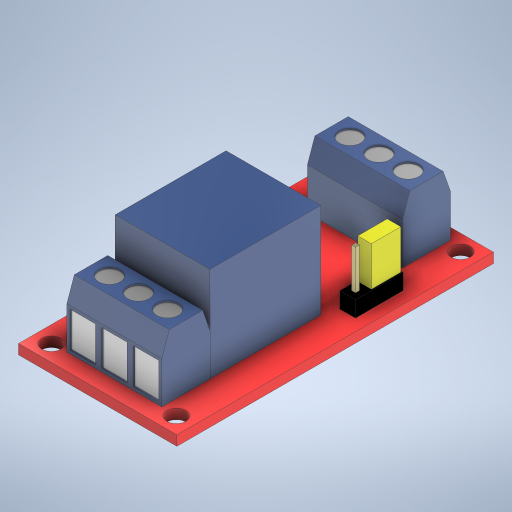
# Autodesk Inventor part: Relay
Saved by Autodesk Inventor 2024 (Build 280153000, 153)
## iProperties
Created: 2023-08-11
Part Number: Relay
Material: Generic
Document SubType Name: Modeling
Designer: 18179
Density: 1 g/cm^3
Appearance: Default
Author: 18179
Autodesk Inventor part; units mm, degrees
ref_plane "YZ Plane" through (0, 0, 0) normal (1, 0, 0) x (0, 1, 0)
ref_plane "XZ Plane" through (0, 0, 0) normal (0, 1, 0) x (-1, 0, 0)
ref_plane "XY Plane" through (0, 0, 0) normal (0, 0, 1) x (1, 0, 0)
sketch "Sketch1" plane through (0, 0, 0) normal (0, 1, 0) x (-1, 0, 0)
  line L0 (0, 0) -> (25.4, 0)
  line L1 (25.4, 0) -> (25.4, -50.8)
  line L2 (25.4, -50.8) -> (0, -50.8)
  line L3 (0, -50.8) -> (0, 0)
  line L4 (25.4, 0) -> (24.257, 0) construction
  line L5 (24.257, 0) -> (24.257, -1.143) construction
  line L6 (24.257, -1.143) -> (25.4, -1.143) construction
  line L7 (25.4, -1.143) -> (25.4, 0) construction
  line L8 (24.257, -1.143) -> (21.209, -1.143) construction
  line L9 (21.209, -1.143) -> (21.209, -4.0275) construction
  line L10 (21.209, -4.0275) -> (24.257, -4.0275) construction
  line L11 (24.257, -4.0275) -> (24.257, -1.143) construction
  line L12 (12.7, 0) -> (12.7, -12.2886) construction
  line L13 (25.4, -25.4) -> (17.1181, -25.4) construction
  circle A0 centre (22.733, -2.5852) radius 1.524
  circle A1 centre (2.667, -2.5852) radius 1.524
  circle A2 centre (22.733, -48.2148) radius 1.524
  circle A3 centre (2.667, -48.2148) radius 1.524
  dimension "d0" = 25.4
  dimension "d1" = 50.8
  dimension "d2" = 1.143
  dimension "d3" = 1.143
  dimension "d4" = 3.048
  constraints: 28 end point, 6 parallel, 4 centre point, 4 horizontal, 3 perpendicular, 3 symmetric about line, 2 midpoint, 1 vertical, 3 other
  measures "d0" distance of L1.end L2.end
  measures "d1" distance of L0.end L1.end
  measures "d2" distance of L6.end L5.end
  measures "d3" distance of L5.end L4.end
  measures "d4" distance of L10.end L9.end
extrude "Extrusion1" add sketch "Sketch1" along normal blind 1.6002
sketch "Sketch3" plane through (0, 1.6002, 0) normal (0, 1, 0) x (1, 0, 0)
  line L0 (0, 50.8) -> (-25.4, 50.8) projected
  line L1 (-12.7, 50.8) -> (-12.7, 49.022)
  line L2 (-12.7, 49.022) -> (-12.7, 41.275)
  line L3 (-25.4, 0) -> (0, 0) projected
  line L4 (-12.7, 0) -> (-12.7, 2.667)
  line L5 (-12.7, 2.667) -> (-12.7, 10.414)
  line L6 (-12.7, 10.414) -> (-5.08, 10.414)
  line L7 (-5.08, 10.414) -> (-20.32, 10.414)
  line L8 (-20.32, 10.414) -> (-20.32, 2.667)
  line L9 (-20.32, 2.667) -> (-5.08, 2.667)
  line L10 (-5.08, 2.667) -> (-5.08, 10.414)
  line L11 (-12.7, 41.275) -> (-5.08, 41.275)
  line L12 (-5.08, 41.275) -> (-5.08, 49.022)
  line L13 (-5.08, 49.022) -> (-12.7, 49.022)
  line L14 (-12.7, 49.022) -> (-12.7, 41.275)
  line L15 (-5.08, 41.275) -> (-20.32, 41.275)
  line L16 (-20.32, 41.275) -> (-20.32, 49.022)
  line L17 (-20.32, 49.022) -> (-5.08, 49.022)
  line L18 (-5.08, 49.022) -> (-5.08, 41.275)
  dimension "d13" = 7.747
  dimension "d14" = 1.778
  dimension "d15" = 2.667
  dimension "d16" = 7.747
  dimension "d17" = 7.62
  dimension "d18" = 15.24
  dimension "d19" = 7.747
  dimension "d20" = 7.62
  dimension "d21" = 7.747
  dimension "d22" = 15.24
  constraints: 34 end point, 6 parallel, 4 perpendicular, 3 horizontal, 3 point on line, 2 midpoint, 2 vertical
  measures "d13" distance of L1.end L2.end
  measures "d14" distance of L1.start L1.end
  measures "d15" distance of L4.start L4.end
  measures "d16" distance of L4.end L5.end
  measures "d17" distance of L5.end L6.end
  measures "d18" distance of L9.end L8.end
  measures "d19" distance of L8.end L7.end
  measures "d20" distance of L13.end L12.end
  measures "d21" distance of L12.end L11.end
  measures "d22" distance of L16.end L17.end
extrude "Extrusion2" add sketch "Sketch3" along normal blind 10.16
chamfer "Chamfer1" distance 1.1938 distance2 3.429 2 edges at (-12.7, 11.7602, -2.667) (-12.7, 11.7602, -10.414) measured on face at (-12.7, 11.7602, -9.914) measured on face at (-12.7, 11.7602, -3.167)
chamfer "Chamfer2" distance 1.1938 distance2 3.429 2 edges at (-12.7, 11.7602, -41.275) (-12.7, 11.7602, -49.022) measured on face at (-12.7, 11.7602, -48.522) measured on face at (-12.7, 11.7602, -41.775)
sketch "Sketch4" plane through (0, 11.7602, 0) normal (0, 1, 0) x (1, 0, 0)
  line L0 (-5.08, 42.4688) -> (-20.32, 42.4688) projected
  line L1 (-20.32, 41.275) -> (-20.32, 49.022) projected
  line L2 (-5.08, 42.4688) -> (-20.32, 42.4688)
  line L3 (-20.32, 42.4688) -> (-20.32, 45.1485)
  line L4 (-20.32, 45.1485) -> (-5.08, 45.1485)
  line L5 (-5.08, 45.1485) -> (-5.08, 42.4688)
  circle A0 centre (-12.7, 45.1485) radius 1.7145
  line L6 (-10.9855, 45.1485) -> (-5.08, 45.1485)
  line L7 (-5.08, 49.022) -> (-5.08, 41.275) projected
  line L8 (-14.4145, 45.1485) -> (-20.32, 45.1485)
  line L9 (-5.08, 3.8608) -> (-20.32, 3.8608) projected
  line L10 (-20.32, 2.667) -> (-20.32, 10.414) projected
  line L11 (-5.08, 3.8608) -> (-20.32, 3.8608)
  line L12 (-20.32, 3.8608) -> (-20.32, 6.5405)
  line L13 (-20.32, 6.5405) -> (-5.08, 6.5405)
  line L14 (-5.08, 6.5405) -> (-5.08, 3.8608)
  circle A1 centre (-8.0328, 45.1485) radius 1.7145
  circle A2 centre (-17.3672, 45.1485) radius 1.7145
  circle A3 centre (-12.7, 6.5405) radius 1.7145
  line L15 (-10.9855, 6.5405) -> (-5.08, 6.5405)
  line L16 (-14.4145, 6.5405) -> (-20.32, 6.5405)
  circle A4 centre (-17.3672, 6.5405) radius 1.7145
  circle A5 centre (-8.0328, 6.5405) radius 1.7145
  point P0 (0, 0)
  dimension "d31" = 3.429
  dimension "d32" = 3.429
  dimension "d33" = 3.429
  dimension "d34" = 3.429
  dimension "d35" = 3.429
  dimension "d36" = 3.429
  constraints: 24 end point, 8 midpoint, 6 centre point, 4 parallel, 4 point on circle, 4 point on line, 3 collinear, 3 perpendicular, 2 horizontal
  measures "d31" diameter of A0
  measures "d32" diameter of A1
  measures "d33" diameter of A2
  measures "d34" diameter of A3
  measures "d35" diameter of A4
  measures "d36" diameter of A5
extrude "Extrusion3" cut sketch "Sketch4" against normal blind 0.254 contours A1 L4 | L4 A1 | A2 L4 | L4 A2 | A0 L4 | L4 A0 | A5 L13 | L13 A5 | A4 L13 | L13 A4 | A3 L13 | L13 A3
sketch "Sketch5" plane through (-20.32, 1.6002, -2.667) normal (0, 0, 1) x (1, 0, 0)
  line L0 (0, 0) -> (0, 6.731) projected
  line L1 (0, 6.731) -> (5.08, 6.731)
  line L2 (15.24, 6.731) -> (0, 6.731) projected
  line L3 (5.08, 6.731) -> (10.16, 6.731)
  line L4 (10.16, 6.731) -> (15.24, 6.731)
  line L5 (10.16, 6.731) -> (15.24, 6.731)
  line L6 (15.24, 6.731) -> (15.24, 0)
  line L7 (15.24, 0) -> (10.16, 0)
  line L8 (10.16, 0) -> (10.16, 6.731)
  line L9 (5.08, 6.731) -> (0, 6.731)
  line L10 (0, 6.731) -> (0, 0)
  line L11 (0, 0) -> (5.08, 0)
  line L12 (5.08, 0) -> (5.08, 6.731)
  line L13 (5.08, 6.731) -> (10.16, 6.731)
  line L14 (10.16, 6.731) -> (10.16, 0)
  line L15 (10.16, 0) -> (5.08, 0)
  line L16 (5.08, 0) -> (5.08, 6.731)
  line L17 (4.572, 6.223) -> (0.508, 6.223)
  line L18 (0.508, 6.223) -> (0.508, 0.508)
  line L19 (0.508, 0.508) -> (4.572, 0.508)
  line L20 (4.572, 0.508) -> (4.572, 6.223)
  line L21 (10.16, 0.508) -> (14.732, 0.508)
  line L22 (14.732, 0.508) -> (14.732, 6.223)
  line L23 (14.732, 6.223) -> (10.16, 6.223)
  line L24 (10.668, 0) -> (10.668, 6.731)
  line L25 (9.652, 0) -> (9.652, 6.223)
  line L26 (9.652, 6.223) -> (5.08, 6.223)
  line L27 (10.16, 0.508) -> (5.588, 0.508)
  line L28 (5.588, 0.508) -> (5.588, 6.731)
  point P0 (20.32, -1.6002)
  point P1 (10.668, 6.223)
  point P2 (10.668, 0.508)
  point P3 (5.588, 6.223)
  point P4 (9.652, 0.508)
  dimension "d39" = 5.08
  dimension "d40" = 5.08
  dimension "d41" = 0.508
  dimension "d42" = 0.508
  dimension "d43" = 0.508
  dimension "d44" = 0.508
  dimension "d45" = 0.508
  constraints: 54 end point, 10 parallel, 6 perpendicular, 3 horizontal, 2 point on line, 1 collinear, 7 other
  measures "d39" distance of L0.end L1.end
  measures "d40" distance of L1.end L3.end
  measures "d41" distance between parallel lines of L12 L20
  measures "d42" distance between parallel lines of L6 L22
  measures "d43" distance between parallel lines of L8 L24
  measures "d44" distance between parallel lines of L14 L25
  measures "d45" distance between parallel lines of L15 L27
extrude "Extrusion4" cut sketch "Sketch5" against normal blind 0.254 contours L26 L25 L27 L28 | L24 L23 L22 L21 | L20 L19 L18 L17
sketch "Sketch6" plane through (-5.08, 1.6002, -49.022) normal (0, 0, -1) x (-1, 0, 0)
  line L0 (0, 0) -> (15.24, 0) projected
  line L1 (15.24, 6.731) -> (0, 6.731) projected
  line L2 (0, 0) -> (5.08, 0)
  line L3 (5.08, 0) -> (5.08, 6.731)
  line L4 (5.08, 6.731) -> (0, 6.731)
  line L5 (0, 6.731) -> (0, 0)
  line L6 (5.08, 6.731) -> (10.16, 6.731)
  line L7 (10.16, 6.731) -> (10.16, 0)
  line L8 (10.16, 0) -> (5.08, 0)
  line L9 (5.08, 0) -> (5.08, 6.731)
  line L10 (15.24, 0) -> (15.24, 6.731) projected
  line L11 (10.16, 0) -> (15.24, 0)
  line L12 (15.24, 0) -> (15.24, 6.731)
  line L13 (15.24, 6.731) -> (10.16, 6.731)
  line L14 (10.16, 6.731) -> (10.16, 0)
  line L15 (0, 6.223) -> (14.732, 6.223)
  line L16 (14.732, 6.223) -> (14.732, 0.508)
  line L17 (14.732, 0.508) -> (0, 0.508)
  line L18 (0.508, 0.508) -> (4.572, 0.508)
  line L19 (4.572, 0.508) -> (4.572, 6.223)
  line L20 (4.572, 6.223) -> (0.508, 6.223)
  line L21 (0.508, 6.223) -> (0.508, 0.508)
  line L22 (9.652, 0) -> (9.652, 6.223)
  line L23 (9.652, 6.223) -> (5.08, 6.223)
  line L24 (10.668, 0.508) -> (14.732, 0.508)
  line L25 (14.732, 0.508) -> (14.732, 6.223)
  line L26 (14.732, 6.223) -> (10.668, 6.223)
  line L27 (10.668, 6.223) -> (10.668, 0.508)
  line L28 (5.588, 7.239) -> (5.588, -0.508)
  line L29 (5.588, -0.508) -> (-0.508, -0.508)
  line L30 (-0.508, -0.508) -> (-0.508, 7.239)
  line L31 (-0.508, 7.239) -> (5.588, 7.239)
  point P0 (-5.08, -1.6002)
  point P1 (5.588, 6.223)
  point P2 (5.588, 0.508)
  point P3 (9.652, 0.508)
  point P4 (0.508, 6.223)
  point P5 (0.508, 0.508)
  dimension "d48" = 5.08
  dimension "d49" = 5.08
  dimension "d50" = 0.508
  dimension "d51" = 0.508
  dimension "d52" = 0.508
  dimension "d53" = 0.508
  dimension "d54" = 0.508
  constraints: 58 end point, 12 parallel, 7 perpendicular, 3 horizontal, 2 point on line, 12 other
  measures "d48" distance of L4.end L3.end
  measures "d49" distance of L7.end L8.end
  measures "d50" distance between parallel lines of L1 L15
  measures "d51" distance between parallel lines of L5 L21
  measures "d52" distance between parallel lines of L7 L22
  measures "d53" distance between parallel lines of L14 L27
  measures "d54" distance between parallel lines of L3 L28
extrude "Extrusion5" cut sketch "Sketch6" against normal blind 0.254 contours L21 L15 L19 L17 | L28 L15 L22 L17 | L27 L15 L16 L17
sketch "Sketch7" plane through (0, 1.6002, 0) normal (0, 1, 0) x (1, 0, 0)
  line L0 (-20.32, 10.414) -> (-5.08, 10.414) projected
  line L1 (-12.7, 10.414) -> (-5.1054, 10.414)
  line L2 (-5.1054, 10.414) -> (-5.1054, 28.194)
  line L3 (-5.1054, 28.194) -> (-12.7, 28.194)
  line L4 (-12.7, 28.194) -> (-12.7, 10.414)
  line L5 (-12.7, 28.194) -> (-20.2946, 28.194)
  line L6 (-20.2946, 28.194) -> (-20.2946, 9.398)
  line L7 (-20.2946, 9.398) -> (-12.7, 9.398)
  line L8 (-12.7, 9.398) -> (-12.7, 28.194)
  point P0 (0, 0)
  point P1 (-20.2946, 10.414)
  dimension "d57" = 7.5946
  dimension "d58" = 17.78
  dimension "d59" = 7.5946
  dimension "d60" = 18.796
  constraints: 16 end point, 4 parallel, 2 horizontal, 2 perpendicular, 1 midpoint
  measures "d57" distance of L3.end L2.end
  measures "d58" distance of L2.end L1.end
  measures "d59" distance of L7.end L6.end
  measures "d60" distance of L6.end L5.end
extrude "Extrusion6" add sketch "Sketch7" along normal blind 15.24 contours L4 L3 L2 L0 | L0 L6 L5 L4
sketch "Sketch8" plane through (0, 1.6002, 0) normal (0, 1, 0) x (1, 0, 0)
  line L0 (-1.8843, 30.5641) -> (-4.4243, 30.5641)
  line L1 (-4.4243, 30.5641) -> (-4.4243, 38.1841)
  line L2 (-4.4243, 38.1841) -> (-1.8843, 38.1841)
  line L3 (-1.8843, 38.1841) -> (-1.8843, 30.5641)
  point P0 (0, 0)
  dimension "d65" = 7.62
  dimension "d66" = 2.54
  constraints: 8 end point, 2 parallel, 1 horizontal, 1 perpendicular
  measures "d65" distance of L2.end L0.start
  measures "d66" distance of L0.start L0.end
extrude "Extrusion7" add sketch "Sketch8" along normal blind 2.54
sketch "Sketch10" plane through (0, 4.1402, 0) normal (0, 1, 0) x (1, 0, 0)
  line L0 (-1.8843, 30.5641) -> (-4.4243, 30.5641) projected
  line L1 (-4.4243, 38.1841) -> (-4.4243, 30.5641) projected
  line L2 (-1.8843, 30.5641) -> (-4.4243, 30.5641)
  line L3 (-4.4243, 30.5641) -> (-4.4243, 35.6441)
  line L4 (-4.4243, 35.6441) -> (-1.8843, 35.6441)
  line L5 (-1.8843, 35.6441) -> (-1.8843, 30.5641)
  line L6 (-1.8843, 35.6441) -> (-4.4243, 35.6441)
  line L7 (-4.4243, 35.6441) -> (-4.4243, 38.1841)
  line L8 (-4.4243, 38.1841) -> (-1.8843, 38.1841)
  line L9 (-1.8843, 38.1841) -> (-1.8843, 35.6441)
  line L10 (-2.8399, 37.2285) -> (-3.4687, 37.2285)
  line L11 (-3.4687, 37.2285) -> (-3.4687, 36.5997)
  line L12 (-3.4687, 36.5997) -> (-2.8399, 36.5997)
  line L13 (-2.8399, 36.5997) -> (-2.8399, 37.2285)
  line L14 (-2.0625, 35.4658) -> (-4.246, 35.4658)
  line L15 (-4.246, 35.4658) -> (-4.246, 30.7423)
  line L16 (-4.246, 30.7423) -> (-2.0625, 30.7423)
  line L17 (-2.0625, 30.7423) -> (-2.0625, 35.4658)
  line L18 (-3.1543, 30.5641) -> (-3.1543, 38.1841)
  line L19 (-3.1543, 34.3741) -> (-3.6306, 34.3741)
  line L20 (-2.8399, 31.5197) -> (-3.4687, 31.5197)
  line L21 (-3.4687, 31.5197) -> (-3.4687, 32.1485)
  line L22 (-3.4687, 32.1485) -> (-2.8399, 32.1485)
  line L23 (-2.8399, 32.1485) -> (-2.8399, 31.5197)
  line L24 (-2.0625, 33.2823) -> (-4.246, 33.2823)
  line L25 (-4.246, 33.2823) -> (-4.246, 38.0058)
  line L26 (-4.246, 38.0058) -> (-2.0625, 38.0058)
  line L27 (-2.0625, 38.0058) -> (-2.0625, 33.2823)
  line L28 (-1.8843, 38.1841) -> (-4.4243, 38.1841) projected
  line L29 (-4.4243, 38.1841) -> (-4.4243, 30.5641) projected
  line L30 (-4.4243, 30.5641) -> (-1.8843, 30.5641) projected
  line L31 (-1.8843, 30.5641) -> (-1.8843, 38.1841) projected
  line L32 (-4.246, 38.0058) -> (-2.0625, 38.0058)
  line L33 (-2.0625, 38.0058) -> (-2.0625, 33.2823)
  line L34 (-2.0625, 33.2823) -> (-4.246, 33.2823)
  line L35 (-4.246, 33.2823) -> (-4.246, 38.0058)
  line L36 (-2.8399, 32.1485) -> (-3.4687, 32.1485)
  line L37 (-3.4687, 32.1485) -> (-3.4687, 31.5197)
  line L38 (-3.4687, 31.5197) -> (-2.8399, 31.5197)
  line L39 (-2.8399, 31.5197) -> (-2.8399, 32.1485)
  point P0 (0, 0)
  dimension "d67" = 5.08
  constraints: 68 end point, 12 parallel, 8 symmetric about line, 6 perpendicular, 5 horizontal, 3 midpoint, 1 point on line, 6 other
  measures "d67" distance of L2.end L3.end
extrude "Extrusion8" add sketch "Sketch10" along normal blind 6.35 contours L27 L14 L18 L4 | L4 L18 L12 L13 L10 L26 L27 | L20 L21 L22 L18 | L18 L22 L23 L20 | L18 L14 L25 L4 | L4 L25 L26 L18 L10 L11 L12 | L17 L24 L18 L14 | L15 L14 L18 L24 | L18 L10 L13 L12 | L12 L11 L10 L18
sketch "Sketch11" plane through (0, 0, 0) normal (0, -1, 0) x (1, 0, 0)
  circle A0 centre (-17.3672, -6.5405) radius 1.7145 projected
  circle A1 centre (-12.7, -6.5405) radius 1.7145 projected
  circle A2 centre (-8.0328, -6.5405) radius 1.7145 projected
  line L0 (-20.2946, -28.194) -> (-20.2946, -10.414) projected
  line L1 (-20.2946, -10.414) -> (-5.1054, -10.414) projected
  line L2 (-5.1054, -10.414) -> (-5.1054, -28.194) projected
  line L3 (-5.1054, -28.194) -> (-20.2946, -28.194) projected
  circle A3 centre (-17.3672, -45.1485) radius 1.7145 projected
  circle A4 centre (-12.7, -45.1485) radius 1.7145 projected
  circle A5 centre (-8.0328, -45.1485) radius 1.7145 projected
  line L4 (-2.8399, -31.5197) -> (-3.4687, -31.5197) projected
  line L5 (-3.4687, -31.5197) -> (-3.4687, -32.1485) projected
  line L6 (-3.4687, -32.1485) -> (-2.8399, -32.1485) projected
  line L7 (-2.8399, -32.1485) -> (-2.8399, -31.5197) projected
  line L8 (-2.0625, -38.0058) -> (-2.0625, -33.2823) projected
  line L9 (-2.0625, -33.2823) -> (-4.246, -33.2823) projected
  line L10 (-4.246, -33.2823) -> (-4.246, -38.0058) projected
  line L11 (-4.246, -38.0058) -> (-2.0625, -38.0058) projected
  line L12 (-1.8843, -38.1841) -> (-4.4243, -38.1841) projected
  line L13 (-4.4243, -38.1841) -> (-4.4243, -30.5641) projected
  line L14 (-4.4243, -30.5641) -> (-1.8843, -30.5641) projected
  line L15 (-1.8843, -30.5641) -> (-1.8843, -38.1841) projected
  circle A6 centre (-8.0328, -6.5405) radius 1.016
  circle A7 centre (-12.7, -6.5405) radius 1.016
  circle A8 centre (-17.3672, -6.5405) radius 1.016
  circle A9 centre (-12.7, -25.6281) radius 1.016
  circle A10 centre (-7.0168, -19.304) radius 1.016
  circle A11 centre (-18.3832, -19.304) radius 1.016
  circle A12 centre (-3.1543, -31.8341) radius 0.635
  circle A13 centre (-3.1543, -36.776) radius 0.635
  circle A14 centre (-3.1543, -34.3741) radius 0.635
  circle A15 centre (-8.0328, -45.1485) radius 1.016
  circle A16 centre (-12.7, -45.1485) radius 1.016
  circle A17 centre (-17.3672, -45.1485) radius 1.016
  point P0 (0, 0)
  dimension "d70" = 2.032
  dimension "d71" = 2.032
  dimension "d72" = 2.032
  dimension "d73" = 2.032
  dimension "d74" = 2.032
  dimension "d75" = 2.032
  dimension "d76" = 1.27
  dimension "d77" = 1.27
  dimension "d78" = 1.27
  dimension "d79" = 2.032
  dimension "d80" = 2.032
  dimension "d81" = 2.032
  constraints: 12 centre point, 6 coincident
  measures "d70" diameter of A6
  measures "d71" diameter of A7
  measures "d72" diameter of A8
  measures "d73" diameter of A9
  measures "d74" diameter of A10
  measures "d75" diameter of A11
  measures "d76" diameter of A12
  measures "d77" diameter of A13
  measures "d78" diameter of A14
  measures "d79" diameter of A15
  measures "d80" diameter of A16
  measures "d81" diameter of A17
extrude "Extrusion9" add sketch "Sketch11" along normal blind 2.032 contours L7 L6 L5 L4 | A6 | A7 | A8 | A9 | A10 | A11 | A12 | A13 | A14 | A15 | A16 | A17
fillet "Fillet1" radius 0.508 12 edges at (-9.0488, -2.032, -6.5405) (-13.716, -2.032, -6.5405) (-18.3832, -2.032, -6.5405) (-8.0328, -2.032, -19.304) (-19.3992, -2.032, -19.304) (-13.716, -2.032, -25.6281) (-3.7893, -2.032, -31.8341) (-3.7893, -2.032, -34.3741) (-3.7893, -2.032, -36.776) (-9.0488, -2.032, -45.1485) (-13.716, -2.032, -45.1485) (-18.3833, -2.032, -45.1485)
body "Solid1"
